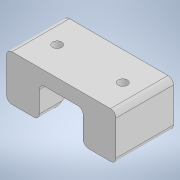
# Autodesk Inventor part: Motor Clamp
Saved by Autodesk Inventor 2022 (Build 260153000, 153)
## iProperties
Created: 2022-08-21
Part Number: Motor Clamp
Material: Generic
Document SubType Name: Modeling
Designer: Nick
Density: 1 g/cm^3
Appearance: Default
Author: Nick
Autodesk Inventor part; units mm, degrees
ref_plane "YZ Plane" through (0, 0, 0) normal (1, 0, 0) x (0, 1, 0)
ref_plane "XZ Plane" through (0, 0, 0) normal (0, 1, 0) x (-1, 0, 0)
ref_plane "XY Plane" through (0, 0, 0) normal (0, 0, 1) x (1, 0, 0)
sketch "Sketch1" plane through (0, 0, 0) normal (0, 0, 1) x (1, 0, 0)
  line L0 (12, 0) -> (12, 11.7)
  line L1 (12, 11.7) -> (28, 11.7)
  line L2 (28, 11.7) -> (28, 0)
  line L3 (28, 0) -> (40, 0)
  line L4 (40, 0) -> (40, 16.7)
  line L5 (40, 16.7) -> (0, 16.7)
  line L6 (0, 16.7) -> (0, 0)
  line L7 (0, 0) -> (12, 0)
  dimension "d0" = 11.7
  dimension "d1" = 16
  dimension "d2" = 12
  dimension "d3" = 12
  dimension "d4" = 5
  constraints: 16 end point, 5 perpendicular, 2 horizontal, 1 coincident, 1 point on line, 1 vertical
  measures "d0" distance of L0.start L0.end
  measures "d1" distance of L0.end L1.end
  measures "d2" distance of L2.end L3.end
  measures "d3" distance of L6.end L0.start
  measures "d4" distance between parallel lines of L1 L5
extrude "Extrusion1" add sketch "Sketch1" along normal blind 21
ref_plane "Work Plane1" through (0, 3, 0) normal (0, -1, 0) x (1, 0, 0)
sketch "Sketch3" plane through (0, 3, 0) normal (0, -1, 0) x (1, 0, 0)
  line L0 (0, 0) -> (12, 0) projected
  line L1 (12, 0) -> (12, 21) projected
  line L2 (0, 21) -> (12, 21) projected
  line L3 (0, 0) -> (0, 21) projected
  line L4 (28, 0) -> (40, 0) projected
  line L5 (40, 0) -> (40, 21) projected
  line L6 (28, 21) -> (40, 21) projected
  line L7 (28, 0) -> (28, 21) projected
  circle A0 centre (8, 10.5) radius 4
  circle A1 centre (32, 10.5) radius 4
  line L8 (8, 10.5) -> (32, 10.5) construction
  line L9 (12, 21) -> (28, 21) construction
  point P0 (20, 21)
  point P1 (20, 10.5)
  point P2 (0, 10.5)
  dimension "d13" = 8
  dimension "d14" = 8
  dimension "d15" = 24
  constraints: 3 midpoint, 2 centre point, 2 end point, 1 horizontal alignment, 1 perpendicular, 1 vertical alignment
  measures "d13" diameter of A0
  measures "d14" diameter of A1
  measures "d15" distance of L8.start L8.end
extrude "Extrusion3" cut sketch "Sketch3" along normal blind 3 draft 30 contours A0 | A1
sketch "Sketch4" plane through (8, 3, 10.5) normal (0, -1, 0) x (1, 0, 0)
  circle A0 centre (0, 0) radius 4 projected
  circle A1 centre (24, 0) radius 4 projected
  point P0 (-8, -10.5)
  point P1 (4, 0)
  point P2 (20, 0)
  constraints: 2 horizontal alignment
hole "Hole1" at (8, 3, 10.5) at (32, 3, 10.5) direction (0, 1, 0) diameter 3.4 end through all clearance for "Flat Head Machine Screw" size "M3" standard "Ansi Metric M Profile"
fillet "Fillet1" radius 2 10 edges at (12, 11.7, 10.5) (28, 11.7, 10.5) (12, 0, 17.8028) (12, 0, 3.1972) (28, 0, 3.1972) (28, 0, 17.8028) (0, 0, 10.5) (40, 0, 10.5) (40, 16.7, 10.5) (0, 16.7, 10.5)
body "Solid1"
